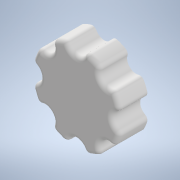
# Autodesk Inventor part: Ручка
Saved by Autodesk Inventor 2020 (Build 240168000, 168)
## iProperties
Created: 2020-12-07
Part Number: Ручка
Material: Типовые
Document SubType Name: Modeling
Designer: User
Density: 1 g/cm^3
Appearance: По умолчанию
Author: User
Autodesk Inventor part; units mm, degrees
ref_plane "YZ Plane" through (0, 0, 0) normal (1, 0, 0) x (0, 1, 0)
ref_plane "XZ Plane" through (0, 0, 0) normal (0, 1, 0) x (-1, 0, 0)
ref_plane "XY Plane" through (0, 0, 0) normal (0, 0, 1) x (1, 0, 0)
sketch "Эскиз1" plane through (0, 0, 0) normal (0, 0, 1) x (1, 0, 0)
  line L0 (-7.0634, 0.5789) -> (-5.187, 3.8289) projected
  line L1 (-5.187, 3.8289) -> (-3.3107, 7.0789) projected
  line L2 (-3.3107, 7.0789) -> (0.4421, 7.0789) projected
  line L3 (0.4421, 7.0789) -> (4.1949, 7.0789) projected
  line L4 (4.1949, 7.0789) -> (6.0713, 3.8289) projected
  line L5 (6.0713, 3.8289) -> (7.9477, 0.5789) projected
  line L6 (7.9477, 0.5789) -> (6.0713, -2.6711) projected
  line L7 (6.0713, -2.6711) -> (4.1949, -5.9211) projected
  line L8 (4.1949, -5.9211) -> (0.4421, -5.9211) projected
  line L9 (0.4421, -5.9211) -> (-3.3107, -5.9211) projected
  line L10 (-3.3107, -5.9211) -> (-5.187, -2.6711) projected
  line L11 (-5.187, -2.6711) -> (-7.0634, 0.5789) projected
  line L12 (0.4421, 7.0789) -> (0.4421, -5.9211) construction
  line L13 (-7.0634, 0.5789) -> (7.9477, 0.5789) construction
  circle A0 centre (0.4421, 0.5789) radius 20
  arc A1 (-19.1579, -3.401) -> (-19.1579, 4.5589) centre (-19.5579, 0.5789) ccw
  arc A2 (-10.6029, -16.0946) -> (-16.2314, -10.4661) centre (-13.7, -13.5632) ccw
  arc A3 (4.4221, -19.0211) -> (-3.5378, -19.0211) centre (0.4421, -19.4211) ccw
  arc A4 (17.1157, -10.4661) -> (11.4872, -16.0946) centre (14.5843, -13.5632) ccw
  arc A5 (20.0421, 4.5589) -> (20.0421, -3.401) centre (20.4421, 0.5789) ccw
  arc A6 (11.4872, 17.2525) -> (17.1157, 11.624) centre (14.5843, 14.7211) ccw
  arc A7 (-3.5378, 20.1789) -> (4.4221, 20.1789) centre (0.4421, 20.5789) ccw
  arc A8 (-16.2314, 11.624) -> (-10.6029, 17.2525) centre (-13.7, 14.7211) ccw
  point P0 (0, 0)
  point P1 (-10.6029, 17.2525)
  point P2 (-16.2314, -10.4661)
  point P3 (-3.5378, -19.0211)
  point P4 (4.4221, -19.0211)
  point P5 (11.4872, -16.0946)
  point P6 (20.0421, -3.401)
  point P7 (20.0421, 4.5589)
  point P8 (17.1157, 11.624)
  point P9 (11.4872, 17.2525)
  point P10 (4.4221, 20.1789)
  point P11 (-3.5378, 20.1789)
  dimension "d0" = 40
  dimension "d1" = 4
  dimension "d4" = 360
  constraints: 19 point on circle, 9 centre point, 4 end point, 1 midpoint, 1 perpendicular, 1 vertical, 33 other
  measures "d0" diameter of A0
  measures "d1" radius of A1
ref_plane "РабПлоскость1" through (-11.9921, -49.7488, -5.3) normal (0, 0, 1) x (0.9986295, -0.052336, 0)
extrude "Выдавливание1" add sketch "Эскиз1" against normal blind 5.8 contours A5 A0 A4 A3 A2 A1 A8 A7 A6
fillet "Сопряжение1" radius 2 16 edges at (-16.2314, -10.4661, -2.9) (-19.1579, -3.401, -2.9) (-19.1579, 4.5589, -2.9) (-16.2314, 11.624, -2.9) (-10.6029, 17.2525, -2.9) (-10.6029, -16.0946, -2.9) (-3.5378, -19.0211, -2.9) (4.4221, -19.0211, -2.9) (11.4872, -16.0946, -2.9) (17.1157, -10.4661, -2.9) (20.0421, -3.401, -2.9) (20.0421, 4.5589, -2.9) (17.1157, 11.624, -2.9) (11.4872, 17.2525, -2.9) (4.4221, 20.1789, -2.9) (-3.5378, 20.1789, -2.9)
sketch "Эскиз2" plane through (0, 0, 0) normal (0, 0, 1) x (1, 0, 0)
  arc A0 (-3.0956, 18.7123) -> (-5.4541, 19.69) centre (-4.8645, 17.7789) ccw projected
  arc A1 (-5.4541, 19.69) -> (-8.9022, 18.2618) centre (0.4421, 0.5789) ccw projected
  arc A2 (-8.9022, 18.2618) -> (-9.8785, 15.9027) centre (-7.9678, 16.4935) ccw projected
  arc A3 (-14.8816, 10.8996) -> (-9.8785, 15.9027) centre (-13.7, 14.7211) ccw projected
  arc A4 (-14.8816, 10.8996) -> (-17.2407, 9.9233) centre (-15.4724, 8.9888) ccw projected
  arc A5 (-17.2407, 9.9233) -> (-18.669, 6.4751) centre (0.4421, 0.5789) ccw projected
  arc A6 (-18.669, 6.4751) -> (-17.6912, 4.1167) centre (-16.7579, 5.8855) ccw projected
  arc A7 (-17.6912, -2.9588) -> (-17.6912, 4.1167) centre (-19.5579, 0.5789) ccw projected
  arc A8 (-17.6912, -2.9588) -> (-18.669, -5.3173) centre (-16.7579, -4.7277) ccw projected
  arc A9 (-18.669, -5.3173) -> (-17.2407, -8.7654) centre (0.4421, 0.5789) ccw projected
  arc A10 (-17.2407, -8.7654) -> (-14.8816, -9.7417) centre (-15.4724, -7.831) ccw projected
  arc A11 (-9.8785, -14.7448) -> (-14.8816, -9.7417) centre (-13.7, -13.5632) ccw projected
  arc A12 (-9.8785, -14.7448) -> (-8.9022, -17.1039) centre (-7.9678, -15.3356) ccw projected
  arc A13 (-8.9022, -17.1039) -> (-5.4541, -18.5322) centre (0.4421, 0.5789) ccw projected
  arc A14 (-5.4541, -18.5322) -> (-3.0956, -17.5544) centre (-4.8645, -16.6211) ccw projected
  arc A15 (3.9799, -17.5544) -> (-3.0956, -17.5544) centre (0.4421, -19.4211) ccw projected
  arc A16 (3.9799, -17.5544) -> (6.3383, -18.5322) centre (5.7487, -16.6211) ccw projected
  arc A17 (6.3383, -18.5322) -> (9.7865, -17.1039) centre (0.4421, 0.5789) ccw projected
  arc A18 (9.7865, -17.1039) -> (10.7628, -14.7448) centre (8.852, -15.3356) ccw projected
  arc A19 (15.7659, -9.7417) -> (10.7628, -14.7448) centre (14.5843, -13.5632) ccw projected
  arc A20 (15.7659, -9.7417) -> (18.125, -8.7654) centre (16.3567, -7.831) ccw projected
  arc A21 (18.125, -8.7654) -> (19.5532, -5.3173) centre (0.4421, 0.5789) ccw projected
  arc A22 (19.5532, -5.3173) -> (18.5755, -2.9588) centre (17.6421, -4.7277) ccw projected
  arc A23 (18.5755, 4.1167) -> (18.5755, -2.9588) centre (20.4421, 0.5789) ccw projected
  arc A24 (18.5755, 4.1167) -> (19.5532, 6.4751) centre (17.6421, 5.8855) ccw projected
  arc A25 (19.5532, 6.4751) -> (18.125, 9.9233) centre (0.4421, 0.5789) ccw projected
  arc A26 (18.125, 9.9233) -> (15.7659, 10.8996) centre (16.3567, 8.9888) ccw projected
  arc A27 (10.7628, 15.9027) -> (15.7659, 10.8996) centre (14.5843, 14.7211) ccw projected
  arc A28 (10.7628, 15.9027) -> (9.7865, 18.2618) centre (8.852, 16.4935) ccw projected
  arc A29 (9.7865, 18.2618) -> (6.3383, 19.69) centre (0.4421, 0.5789) ccw projected
  arc A30 (6.3383, 19.69) -> (3.9799, 18.7123) centre (5.7487, 17.7789) ccw projected
  arc A31 (-3.0956, 18.7123) -> (3.9799, 18.7123) centre (0.4421, 20.5789) ccw projected
  line L0 (7.9477, 0.5789) -> (4.1949, -5.9211) projected
  line L1 (4.1949, -5.9211) -> (-3.3107, -5.9211) projected
  line L2 (-3.3107, -5.9211) -> (-7.0634, 0.5789) projected
  line L3 (-7.0634, 0.5789) -> (-3.3107, 7.0789) projected
  line L4 (-3.3107, 7.0789) -> (4.1949, 7.0789) projected
  line L5 (4.1949, 7.0789) -> (7.9477, 0.5789) projected
  point P0 (0, 0)
extrude "Выдавливание2" add sketch "Эскиз2" along normal blind 7 contours A31 A30 A29 A28 A27 A26 A25 A24 A23 A22 A21 A20 A19 A18 A17 A16 A15 A14 A13 A12 A11 A10 A9 A8 A7 A6 A5 A4 A3 A2 A1 A0 | L0 L1 L2 L3 L4 L5
fillet "Сопряжение2" radius 2 32 edges at (-7.2115, 19.0565, 7) (-9.8158, 17.2583, 7) (-10.8716, 11.8926, 7) (-16.2372, 10.8368, 7) (-18.0355, 8.2326, 7) (-18.6054, 5.1196, 7) (-15.5579, 0.5789, 7) (-18.6054, -3.9617, 7) (-18.0355, -7.0747, 7) (-16.2372, -9.679, 7) (-10.8716, -10.7348, 7) (-9.8158, -16.1004, 7) (-7.2115, -17.8987, 7) (-4.0985, -18.4686, 7) (0.4421, -15.4211, 7) (4.9828, -18.4686, 7) (8.0958, -17.8987, 7) (10.7, -16.1004, 7) (11.7558, -10.7348, 7) (17.1215, -9.679, 7) (18.9197, -7.0747, 7) (19.4896, -3.9617, 7) (16.4421, 0.5789, 7) (19.4896, 5.1196, 7) (18.9197, 8.2326, 7) (17.1215, 10.8368, 7) (11.7558, 11.8926, 7) (10.7, 17.2583, 7) (8.0958, 19.0565, 7) (4.9828, 19.6264, 7) (0.4421, 16.5789, 7) (-4.0985, 19.6264, 7)
